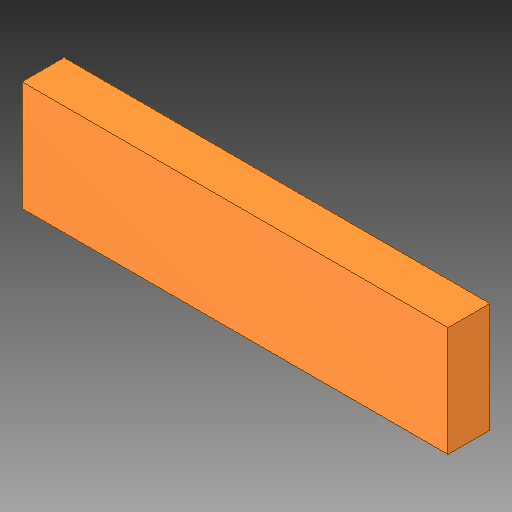
# Autodesk Inventor part: JP2_1X04SMD
Saved by Autodesk Inventor 2017 (Build 210142000, 142)
## iProperties
Created: 2019-06-13
Part Number: JP2_1X04SMD
Material: Generic
Document SubType Name: Modeling
Designer: Marc
Density: 1 g/cm^3
Appearance: 1X04SMD, JP2_1X04SMD
Author: Marc
Autodesk Inventor part; units mm, degrees
ref_plane "YZ Plane" through (0, 0, 0) normal (1, 0, 0) x (0, 1, 0)
ref_plane "XZ Plane" through (0, 0, 0) normal (0, 1, 0) x (-1, 0, 0)
ref_plane "XY Plane" through (0, 0, 0) normal (0, 0, 1) x (1, 0, 0)
sketch "1X04SMD, JP2_1X04SMD_29" plane through (0, 0, 0) normal (0, 0, 1) x (1, 0, 0)
  line L0 (-2.54, 1.3462) -> (7.62, 1.3462)
  line L1 (7.62, 1.3462) -> (7.62, -1.27)
  line L2 (7.62, -1.27) -> (-2.54, -1.27)
  line L3 (-2.54, -1.27) -> (-2.54, 1.3462)
  constraints: 8 end point
extrude "Extrusion1" add sketch "1X04SMD, JP2_1X04SMD_29" along normal blind 1
body "Solid1"
